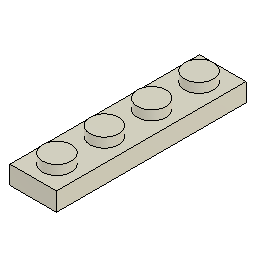
R4xC1xT3_1-VER2 (Autodesk Fusion 360 design; units mm, degrees)
Autodesk Fusion 360 part; units mm, degrees
sketch "Sketch1" plane through (0, 0, 0) normal (0, 0, 1) x (1, 0, 0)
  line L0 (0, 0) -> (7.8, 0)
  line L1 (7.8, 0) -> (7.8, 31.8)
  line L2 (7.8, 31.8) -> (0, 31.8)
  line L3 (0, 31.8) -> (0, 0)
  dimension "d1" = 7.8
  dimension "d2" = 31.8
  constraint horizontal L0
  constraint vertical L1
  constraint horizontal L2
  constraint vertical L3
  constraint coincident L0.start L3.end
  measures "d1" distance of L1.end L2.end
  measures "d2" distance of L0.end L1.end
extrude "Extrude1" add sketch "Sketch1" along normal blind 3.1
sketch "Sketch2" plane through (0, 0, 0) normal (0, 0, -1) x (1, 0, 0)
  line L0 (0, 0) -> (0, -31.8)
  line L1 (0, -31.8) -> (7.8, -31.8)
  line L2 (7.8, -31.8) -> (7.8, 0)
  line L3 (7.8, 0) -> (0, 0)
  line L4 (1.2, -1.2) -> (6.6, -1.2)
  line L5 (6.6, -1.2) -> (6.6, -30.6)
  line L6 (6.6, -30.6) -> (1.2, -30.6)
  line L7 (1.2, -30.6) -> (1.2, -1.2)
  line L8 (-5, -7.95) -> (12, -7.95) construction
  line L9 (-5, -15.9) -> (12, -15.9) construction
  line L10 (-5, -23.85) -> (12, -23.85) construction
  line L11 (1.2, -6.6) -> (6.6, -6.6)
  line L12 (1.2, -9.3) -> (6.6, -9.3)
  line L13 (1.2, -14.55) -> (6.6, -14.55)
  line L14 (1.2, -17.25) -> (6.6, -17.25)
  line L15 (1.2, -22.5) -> (6.6, -22.5)
  line L16 (1.2, -25.2) -> (6.6, -25.2)
  dimension "d5" = 1.2
  dimension "d6" = 1.2
  dimension "d7" = 1.2
  dimension "d8" = 1.2
  dimension "d38" = 7.95
  dimension "d39" = 7.95
  dimension "d40" = 7.95
  dimension "d41" = 1.35
  dimension "d42" = 2.7
  dimension "d43" = 1.35
  dimension "d44" = 2.7
  dimension "d45" = 1.35
  dimension "d46" = 2.7
  constraint horizontal L4
  constraint vertical L5
  constraint horizontal L6
  constraint vertical L7
  constraint perpendicular L7 L8
  constraint perpendicular L2 L9
  constraint perpendicular L2 L10
  constraint coincident L7 L11.start
  constraint coincident L5 L11.end
  constraint perpendicular L5 L11
  constraint coincident L7 L12.start
  constraint coincident L5 L12.end
  constraint perpendicular L5 L12
  constraint coincident L5 L13.end
  constraint perpendicular L5 L13
  constraint coincident L7 L14.start
  constraint coincident L5 L14.end
  constraint perpendicular L5 L14
  constraint coincident L7 L15.start
  constraint coincident L5 L15.end
  constraint perpendicular L5 L15
  constraint coincident L5 L16.end
  constraint perpendicular L5 L16
  constraint coincident L7 L13.start
  constraint coincident L7 L16.start
  measures "d5" distance of L0 L7
  measures "d6" distance of L3 L4
  measures "d7" distance of L1 L6
  measures "d8" distance of L2 L5
  measures "d38" distance of L3 L8
  measures "d39" distance of L8 L9
  measures "d40" distance of L9 L10
  measures "d41" distance of L10 L16
  measures "d42" distance of L15 L16
  measures "d43" distance of L9 L14
  measures "d44" distance of L13 L14
  measures "d45" distance of L8 L12
  measures "d46" distance of L11 L12
sketch "Sketch3" plane through (0, 0, 3.1) normal (0, 0, 1) x (-1, 0, 0)
  line L0 (0, -31.8) -> (0, 0)
  line L1 (0, 0) -> (-7.8, 0)
  line L2 (-7.8, 0) -> (-7.8, -31.8)
  line L3 (-7.8, -31.8) -> (0, -31.8)
  circle A0 centre (-3.9, -27.825) radius 2.4
  circle A1 centre (-3.9, -19.875) radius 2.4
  circle A2 centre (-3.9, -11.925) radius 2.4
  circle A3 centre (-3.9, -3.975) radius 2.4
  dimension "d11" = 4.8
  dimension "d12" = 4.8
  dimension "d13" = 4.8
  dimension "d14" = 4.8
  dimension "d15" = 3.9
  dimension "d16" = 7.95
  dimension "d17" = 7.95
  dimension "d18" = 7.95
  dimension "d19" = 3.975
  dimension "d37" = 3.9
  constraint collinear A1.centre A2.centre A3.centre
  constraint collinear A0.centre A1.centre A2.centre
  measures "d11" diameter of A0
  measures "d12" diameter of A1
  measures "d13" diameter of A2
  measures "d14" diameter of A3
  measures "d15" distance of L0 A0.centre
  measures "d16" vertical distance of A2.centre A3.centre
  measures "d17" vertical distance of A1.centre A2.centre
  measures "d18" vertical distance of A0.centre A1.centre
  measures "d19" distance of L1 A3.centre
  measures "d37" distance of L0 A3.centre
extrude "Extrude3" add sketch "Sketch3" along normal blind 1.6 contours A0 | A1 | A2 | A3
extrude "Extrude6" cut sketch "Sketch2" against normal blind 2 contours L4 L5 L7 L11 | L5 L7 L12 L13 | L5 L7 L14 L15 | L5 L6 L7 L16
